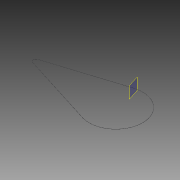
# Autodesk Inventor part: string
Saved by Autodesk Inventor 2013 (Build 170138000, 138)
## iProperties
Created: 2013-10-18
Part Number: string
Material: Generic
Document SubType Name: Modeling
Designer: employee
Density: 1 g/cm^3
Mass: 0.095657 g
Surface Area: 7.65256 cm^2
Volume: 0.095657 cm^3
Author: employee
Autodesk Inventor part; units mm, degrees
ref_plane "YZ Plane" through (0, 0, 0) normal (1, 0, 0) x (0, 1, 0)
ref_plane "XZ Plane" through (0, 0, 0) normal (0, 1, 0) x (-1, 0, 0)
ref_plane "XY Plane" through (0, 0, 0) normal (0, 0, 1) x (1, 0, 0)
sketch "Sketch1" plane through (0, 0, 0) normal (0, 0, 1) x (1, 0, 0)
  arc A0 (-1.5375, 4.8889) -> (-1.5375, -4.8889) centre (0, 0) ccw
  arc A1 (134.9625, -47.8162) -> (134.9625, 47.8162) centre (150, 0) ccw
  line L0 (134.9625, 47.8162) -> (-1.5375, 4.8889)
  line L1 (-1.5375, -4.8889) -> (134.9625, -47.8162)
  dimension "d0" = 150
  dimension "d1" = 10.25
  dimension "d2" = 100.25
  constraints: 4 end point, 4 point on circle, 4 tangent, 2 centre point, 1 coincident, 1 horizontal alignment
  measures "d0" distance of A1.centre point (0, 0)
  measures "d1" diameter of A0
  measures "d2" diameter of A1
ref_plane "Work Plane1" through (134.9625, 47.8162, 0) normal (-0.9539, -0.3, 0) x (0.3, -0.9539, 0)
sketch "Sketch2" plane through (134.9625, 47.8162, 0) normal (-0.9539, -0.3, 0) x (0.3, -0.9539, 0)
  circle A0 centre (0, 0) radius 0.25
  point P0 (5.125, 0)
  dimension "d3" = 0.5
  constraints: 1 centre point, 1 coincident
  measures "d3" diameter of A0
sweep "Sweep1" add profiles "Sketch2" path "Sketch1"
body "Solid1"
